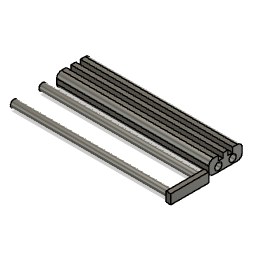
orugaconencastre (Autodesk Fusion 360 design; units mm, degrees)
Autodesk Fusion 360 part; units mm, degrees
sketch "Boceto1" plane through (0, 0, 0) normal (0, 0, 1) x (1, 0, 0)
  line L0 (0, 0) -> (32, 0)
  line L1 (32, 0) -> (32, 7)
  line L2 (32, 7) -> (0, 7)
  line L3 (0, 7) -> (0, 0)
  constraint horizontal L0
  constraint vertical L1
  constraint horizontal L2
  constraint vertical L3
  constraint coincident L0.start L3.end
extrude "Extruir1" add sketch "Boceto1" along normal blind 3 makes body 1
move_body "Desplazar1" bodies 1 to x (1, 0, 0) y (0, 0, 1) z (0, -1, 0) at (0, 0, 0)
move_body "Desplazar2" bodies 1 to x (1, 0, 0) y (0, 1, 0) z (0, 0, 1) at (0, 6, 0)
fillet "Empalme1" radius 1 4 edges at (16, 6, 7) (16, 6, 0) (16, 3, 7) (16, 3, 0) on bodies 1
sketch "Boceto2" plane through (0, 6, 0) normal (0, 1, 0) x (-1, 0, 0)
  line L0 (-32, 1) -> (0, 1)
  line L1 (0, 1) -> (0, 6)
  line L2 (0, 6) -> (-32, 6)
  line L3 (-32, 6) -> (-32, 1)
  line L4 (0, 2) -> (-32, 2)
  line L5 (-32, 2) -> (-32, 3)
  line L6 (-32, 3) -> (0, 3)
  line L7 (0, 3) -> (0, 2)
  line L8 (-32, 4) -> (0, 4)
  line L9 (0, 4) -> (0, 5)
  line L10 (0, 5) -> (-32, 5)
  line L11 (-32, 5) -> (-32, 4)
  constraint horizontal L4
  constraint vertical L5
  constraint horizontal L6
  constraint vertical L7
  constraint coincident L3 L5.end
  constraint coincident L1 L4.start
  constraint horizontal L8
  constraint vertical L9
  constraint horizontal L10
  constraint vertical L11
  constraint coincident L1 L9.end
  constraint coincident L3 L8.start
extrude "Extruir2" cut sketch "Boceto2" against normal blind 1 contours L1 L3 L4 L5 L6 L7 | L1 L3 L8 L9 L10 L11 bodies 1
sketch "Boceto3" plane through (0, 0, 0) normal (-1, 0, 0) x (0, 0, 1)
  line L0 (3, 6) -> (3, 5)
  line L1 (3, 5) -> (2, 5)
  line L2 (2, 5) -> (2, 6)
  line L3 (2, 6) -> (1, 6)
  arc A0 (1, 6) -> (0, 5) centre (1, 5) ccw
  line L4 (0, 5) -> (0, 4)
  arc A1 (0, 4) -> (1, 3) centre (1, 4) ccw
  line L5 (1, 3) -> (6, 3)
  arc A2 (6, 3) -> (7, 4) centre (6, 4) ccw
  line L6 (7, 4) -> (7, 5)
  arc A3 (7, 5) -> (6, 6) centre (6, 5) ccw
  line L7 (6, 6) -> (5, 6)
  line L8 (5, 6) -> (5, 5)
  line L9 (5, 5) -> (4, 5)
  line L10 (4, 5) -> (4, 6)
  line L11 (4, 6) -> (3, 6)
  circle A4 centre (2, 4) radius 0.75
  circle A5 centre (5, 4) radius 0.75
  dimension "d7" = 1.5
  dimension "d8" = 1.5
  measures "d7" diameter of A4
  measures "d8" diameter of A5
extrude "Extruir3" cut sketch "Boceto3" against normal blind 32 contours A4 | A5 bodies 1
sketch "Boceto4" plane through (0, 0, 0) normal (1, 0, 0) x (0, 0, -1)
sketch "Boceto5" plane through (32, 0, 0) normal (1, 0, 0) x (0, 0, -1)
  circle A0 centre (-2, 4) radius 0.75
  circle A1 centre (-5, 4) radius 0.75
  line L0 (-3, 5) -> (-3, 6)
  line L1 (-3, 6) -> (-4, 6)
  line L2 (-4, 6) -> (-4, 5)
  line L3 (-4, 5) -> (-5, 5)
  line L4 (-5, 5) -> (-5, 6)
  line L5 (-5, 6) -> (-6, 6)
  arc A2 (-6, 6) -> (-7, 5) centre (-6, 5) ccw
  line L6 (-7, 5) -> (-7, 4)
  arc A3 (-7, 4) -> (-6, 3) centre (-6, 4) ccw
  line L7 (-6, 3) -> (-1, 3)
  arc A4 (-1, 3) -> (0, 4) centre (-1, 4) ccw
  line L8 (0, 4) -> (0, 5)
  arc A5 (0, 5) -> (-1, 6) centre (-1, 5) ccw
  line L9 (-1, 6) -> (-2, 6)
  line L10 (-2, 6) -> (-2, 5)
  line L11 (-2, 5) -> (-3, 5)
  line L12 (-7.9638, 5) -> (-16.0094, 5)
  line L13 (-16.0094, 5) -> (-16.0094, 3)
  line L14 (-16.0094, 3) -> (-7.9638, 3)
  line L15 (-7.9638, 3) -> (-7.9638, 5)
  line L16 (-12, 4) -> (-15, 4)
  circle A6 centre (-15, 4) radius 0.75
  line L17 (-11.9866, 5) -> (-11.9866, 3)
  circle A7 centre (-8.9732, 4) radius 0.75
  dimension "d11" = 3
  dimension "d12" = 1.5
  constraint horizontal L12
  constraint vertical L13
  constraint horizontal L14
  constraint vertical L15
  constraint parallel L12 L16
  constraint coincident L16.end A6.centre
  constraint midpoint L12 L17.start
  constraint perpendicular L12 L17
  constraint symmetric A6 L17 A7
  measures "d11" distance of L16.start L16.end
  measures "d12" diameter of A6
extrude "Extruir4" add sketch "Boceto5" against normal blind 33 separate body contours A6 | A7 makes body 2 at (10, 3.9253, 8.2269) makes body 3 at (10, 3.9253, 14.2537)
sketch "Boceto6" plane through (32, 0, 0) normal (1, 0, 0) x (0, 0, -1)
  circle A0 centre (-2, 4) radius 0.75
  circle A1 centre (-5, 4) radius 0.75
  line L0 (-3, 5) -> (-3, 6)
  line L1 (-3, 6) -> (-4, 6)
  line L2 (-4, 6) -> (-4, 5)
  line L3 (-4, 5) -> (-5, 5)
  line L4 (-5, 5) -> (-5, 6)
  line L5 (-5, 6) -> (-6, 6)
  arc A2 (-6, 6) -> (-7, 5) centre (-6, 5) ccw
  line L6 (-7, 5) -> (-7, 4)
  arc A3 (-7, 4) -> (-6, 3) centre (-6, 4) ccw
  line L7 (-6, 3) -> (-1, 3)
  arc A4 (-1, 3) -> (0, 4) centre (-1, 4) ccw
  line L8 (0, 4) -> (0, 5)
  arc A5 (0, 5) -> (-1, 6) centre (-1, 5) ccw
  line L9 (-1, 6) -> (-2, 6)
  line L10 (-2, 6) -> (-2, 5)
  line L11 (-2, 5) -> (-3, 5)
  line L12 (-8, 5) -> (-16, 5)
  line L13 (-16, 5) -> (-16, 3)
  line L14 (-16, 3) -> (-8, 3)
  line L15 (-8, 3) -> (-8, 5)
  constraint horizontal L12
  constraint vertical L13
  constraint horizontal L14
  constraint vertical L15
extrude "Extruir5" add sketch "Boceto6" along normal blind 1 contours L12 L13 L14 L15 bodies 2 3
